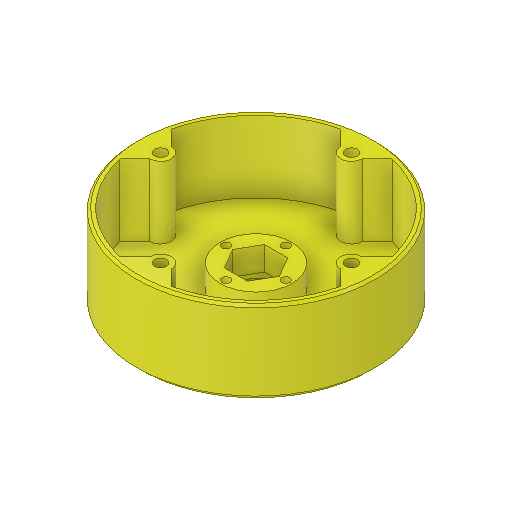
# Autodesk Inventor part: ground_support_0
Saved by Autodesk Inventor 2022 (Build 260153000, 153)
## iProperties
Created: 2019-12-20
Part Number: ground_support_0
Material: Generic
Document SubType Name: Modeling
Designer: nnico
Density: 1 g/cm^3
Appearance: Yellow
Author: nnico
Autodesk Inventor part; units mm, degrees
ref_plane "YZ Plane" through (0, 0, 0) normal (1, 0, 0) x (0, 1, 0)
ref_plane "XZ Plane" through (0, 0, 0) normal (0, 1, 0) x (-1, 0, 0)
ref_plane "XY Plane" through (0, 0, 0) normal (0, 0, 1) x (1, 0, 0)
sketch "Sketch5" plane through (0, 0, 0) normal (0, 1, 0) x (-1, 0, 0)
  circle A0 centre (0, 0) radius 50
  dimension "d10" = 100
  constraints: 1 centre point, 1 coincident
  measures "d10" diameter of A0
extrude "Extrusion4" add sketch "Sketch5" along normal blind 5
sketch "Sketch6" plane through (0, 5, 0) normal (0, 1, 0) x (1, 0, 0)
  circle A0 centre (0, 0) radius 6.25
  dimension "d13" = 12.5
  constraints: 1 centre point, 1 coincident
  measures "d13" diameter of A0
extrude "Extrusion5" cut sketch "Sketch6" against normal blind 5
sketch "Sketch7" plane through (0, 5, 0) normal (0, 1, 0) x (1, 0, 0)
  circle A0 centre (0, 0) radius 50 construction
  line L0 (9.75, 0) -> (4.875, -8.4437)
  line L1 (4.875, -8.4437) -> (-4.875, -8.4437)
  line L2 (-4.875, -8.4437) -> (-9.75, 0)
  line L3 (-9.75, 0) -> (-4.875, 8.4437)
  line L4 (-4.875, 8.4437) -> (4.875, 8.4437)
  line L5 (4.875, 8.4437) -> (9.75, 0)
  line L6 (0, 0) -> (50, 0) construction
  circle A1 centre (0, 0) radius 15
  dimension "d20" = 19.5
  dimension "d21" = 30
  constraints: 14 end point, 2 coincident, 1 centre point, 1 horizontal, 1 horizontal alignment, 1 point on line, 14 other
  measures "d20" distance of L0.start L2.end
  measures "d21" diameter of A1
extrude "Extrusion6" add sketch "Sketch7" along normal blind 10
sketch "Sketch8" plane through (0, 15, 0) normal (0, 1, 0) x (1, 0, 0)
  circle A0 centre (0, 0) radius 12.5 construction
  line L0 (0, 12.5) -> (0, -12.5) construction
  line L1 (-12.5, 0) -> (12.5, 0) construction
  circle A1 centre (0, 12.5) radius 1.75
  circle A2 centre (-12.5, 0) radius 1.75
  circle A3 centre (0, -12.5) radius 1.75
  circle A4 centre (12.5, 0) radius 1.75
  dimension "d24" = 25
  dimension "d25" = 3.5
  dimension "d26" = 3.5
  dimension "d27" = 3.5
  dimension "d28" = 3.5
  constraints: 8 coincident, 5 centre point, 4 end point, 4 midpoint, 4 point on circle, 1 perpendicular, 1 vertical
  measures "d24" diameter of A0
  measures "d25" diameter of A1
  measures "d26" diameter of A2
  measures "d27" diameter of A3
  measures "d28" diameter of A4
extrude "Extrusion7" cut sketch "Sketch8" against normal blind 5
sketch "Sketch9" plane through (0, 5, 0) normal (0, 1, 0) x (1, 0, 0)
  circle A0 centre (0, 0) radius 50
  circle A1 centre (0, 0) radius 47.5
  dimension "d31" = 95
  constraints: 2 centre point, 2 coincident
  measures "d31" diameter of A1
extrude "Extrusion8" add sketch "Sketch9" along normal blind 30
sketch "Sketch10" plane through (0, 5, 0) normal (0, 1, 0) x (1, 0, 0)
  circle A0 centre (0, 0) radius 40 construction
  line L0 (40, 0) -> (-40, 0) construction
  line L1 (0, 40) -> (0, -40) construction
  circle A1 centre (40, 0) radius 4.5
  circle A2 centre (0, 40) radius 4.5
  circle A3 centre (0, -40) radius 4.5
  circle A4 centre (-40, 0) radius 4.5
  dimension "d34" = 80
  dimension "d35" = 9
  dimension "d36" = 9
  dimension "d37" = 9
  dimension "d38" = 9
  constraints: 5 centre point, 5 coincident, 4 end point, 4 point on circle, 3 midpoint, 1 horizontal, 1 perpendicular
  measures "d34" diameter of A0
  measures "d35" diameter of A1
  measures "d36" diameter of A2
  measures "d37" diameter of A3
  measures "d38" diameter of A4
extrude "Extrusion9" add sketch "Sketch10" along normal blind 30
sketch "Sketch11" plane through (40, 35, 0) normal (0, 1, 0) x (1, 0, 0)
  circle A0 centre (0, 0) radius 2.5
  point P0 (-40, 0)
  dimension "d41" = 5
  constraints: 1 centre point
  measures "d41" diameter of A0
extrude "Extrusion10" cut sketch "Sketch11" against normal blind 20
sketch "Sketch12" plane through (0, 35, -40) normal (0, 1, 0) x (1, 0, 0)
  circle A0 centre (0, 0) radius 2.5
  point P0 (0, -40)
  dimension "d44" = 5
  constraints: 1 centre point
  measures "d44" diameter of A0
extrude "Extrusion11" cut sketch "Sketch12" against normal blind 20
sketch "Sketch13" plane through (-40, 35, 0) normal (0, 1, 0) x (1, 0, 0)
  circle A0 centre (0, 0) radius 2.5
  point P0 (40, 0)
  dimension "d47" = 5
  constraints: 1 centre point
  measures "d47" diameter of A0
extrude "Extrusion12" cut sketch "Sketch13" against normal blind 20
sketch "Sketch14" plane through (0, 35, 40) normal (0, 1, 0) x (1, 0, 0)
  circle A0 centre (0, 0) radius 2.5
  point P0 (0, 40)
  dimension "d50" = 5
  constraints: 1 centre point
  measures "d50" diameter of A0
extrude "Extrusion13" cut sketch "Sketch14" against normal blind 20
sketch "Sketch16" plane through (0, 5, 0) normal (0, 1, 0) x (1, 0, 0)
  circle A0 centre (0, 0) radius 47.5 construction
  line L0 (0, 47.5) -> (0, -47.5) construction
  line L1 (-47.5, 0) -> (47.5, 0) construction
  circle A1 centre (-40, 0) radius 2.5 construction
  circle A2 centre (-40, 0) radius 4.5 construction
  circle A3 centre (-40, 0) radius 4.5 construction
  line L2 (-40, 4.5) -> (-40, -4.5) construction
  circle A4 centre (0, 0) radius 47.5 construction
  line L3 (-40, 4.5) -> (-46.2643, 10.7643)
  line L4 (-40, 4.5) -> (-31.141, 4.5) construction
  line L5 (-40, -4.5) -> (-46.2643, -10.7643)
  arc A5 (-46.2643, 10.7643) -> (-46.2643, -10.7643) centre (0, 0) ccw
  arc A6 (-40, 4.5) -> (-40, -4.5) centre (-40, 0) ccw
  circle A7 centre (0, 0) radius 47.5 construction
  circle A8 centre (40, 0) radius 4.5 construction
  circle A9 centre (0, 0) radius 47.5 construction
  line L6 (40, 4.5) -> (46.2643, 10.7643)
  line L7 (40, -4.5) -> (46.2643, -10.7643)
  arc A10 (46.2643, -10.7643) -> (46.2643, 10.7643) centre (0, 0) ccw
  arc A11 (40, -4.5) -> (40, 4.5) centre (40, 0) ccw
  circle A12 centre (0, -40) radius 2.5 construction
  circle A13 centre (0, -40) radius 4.5 construction
  circle A14 centre (0, -40) radius 4.5 construction
  line L8 (4.5, -40) -> (-4.5, -40) construction
  line L9 (-4.5, -40) -> (-10.7643, -46.2643)
  line L10 (4.5, -40) -> (10.7643, -46.2643)
  arc A15 (-10.7643, -46.2643) -> (10.7643, -46.2643) centre (0, 0) ccw
  arc A16 (-4.5, -40) -> (4.5, -40) centre (0, -40) ccw
  line L11 (-4.5, 40) -> (-10.7643, 46.2643)
  line L12 (4.5, 40) -> (10.7643, 46.2643)
  arc A17 (10.7643, 46.2643) -> (-10.7643, 46.2643) centre (0, 0) ccw
  arc A18 (4.5, 40) -> (-4.5, 40) centre (0, 40) ccw
  dimension "d54" = 135
  constraints: 26 end point, 26 point on circle, 12 symmetric about line, 11 centre point, 4 coincident, 3 horizontal, 2 midpoint, 1 equal length, 1 line through centre, 1 perpendicular, 1 tangent, 1 vertical, 14 other
  measures "d54" angle of L4 L3
extrude "Extrusion14" add sketch "Sketch16" along normal blind 30
chamfer "Chamfer1" distance 1 angle 45 1 edges at (-50, 35, 0)
chamfer "Chamfer2" distance 2 angle 45 1 edges at (50, 0, 0)
body "Solid2"
